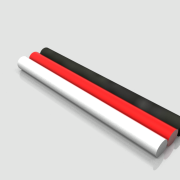
# Autodesk Inventor part: 3-Wire Motor Cable-Cut
Saved by Autodesk Inventor 2013 (Build 170138000, 138)
## iProperties
Category: 3-Wire Motors
Company: Super Sonic Sparks, Team 24
Material: Copper
Catalog Web Link: vexrobotics.com/276-2162.html
Description: Cable of the 3-wire motors.
Vendor: VEX Robotics, Inc.
Document SubType Name: Modeling
Designer: Jordan Kiesel
Mass: 1.02752 g
Surface Area: 2.9937 cm^2
Volume: 0.114936 cm^3
Density: 8.94 g/cm^3
Title: 3-Wire Motor Cable-Cut
Author: Jordan Kiesel
Comments: The cable of the 3-wire motors.
Autodesk Inventor part; units mm, degrees
ref_plane "YZ Plane" through (0, 0, 0) normal (1, 0, 0) x (0, 1, 0)
ref_plane "XZ Plane" through (0, 0, 0) normal (0, 1, 0) x (-1, 0, 0)
ref_plane "XY Plane" through (0, 0, 0) normal (0, 0, 1) x (1, 0, 0)
sketch "Sketch1" plane through (0, 0, 0) normal (1, 0, 0) x (0, 1, 0)
  circle A0 centre (0, 0) radius 0.8001
  dimension "d0" = 1.6002
  constraints: 1 centre point
  measures "d0" diameter of A0
extrude "Extrusion1" add sketch "Sketch1" along normal blind 19.05
sketch "Sketch2" plane through (19.05, 0, 0) normal (1, 0, 0) x (0, 0, -1)
  circle A0 centre (1.6002, 0) radius 0.8001
  circle A1 centre (0, 0) radius 0.8001 projected
  dimension "d3" = 1.6002
  constraints: 1 centre point, 1 equal radius, 1 horizontal alignment
  measures "d3" diameter of A0
extrude "Extrusion2" add sketch "Sketch2" against normal blind 19.05 contours A0
sketch "Sketch3" plane through (19.05, 0, -1.6002) normal (1, 0, 0) x (0, 0, -1)
  circle A0 centre (1.6002, 0) radius 0.8001
  circle A1 centre (0, 0) radius 0.8001 projected
  point P0 (-0.8001, 0)
  dimension "d6" = 1.6002
  constraints: 2 horizontal alignment, 1 centre point, 1 other
  measures "d6" diameter of A0
extrude "Extrusion3" add sketch "Sketch3" against normal blind 19.05 contours A0
body "Solid1"
